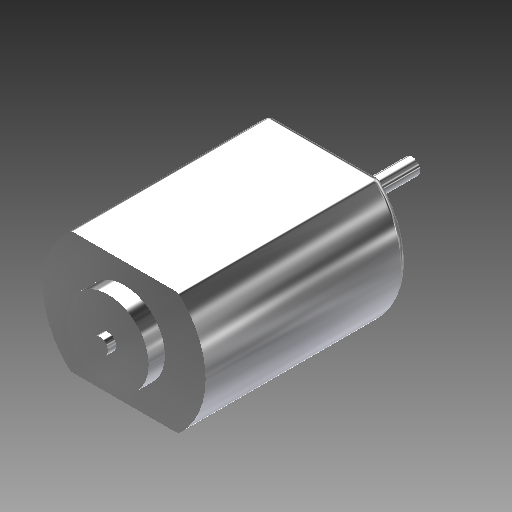
# Autodesk Inventor part: motor
Saved by Autodesk Inventor 2017 (Build 210142000, 142)
## iProperties
Created: 2016-09-08
Part Number: motor
Material: Aluminum 6061
Document SubType Name: Modeling
Designer: Paulo Loma
Density: 2.7 g/cm^3
Appearance: Aluminum - Flat
Author: Paulo Loma
Autodesk Inventor part; units mm, degrees
ref_plane "YZ Plane" through (0, 0, 0) normal (1, 0, 0) x (0, 1, 0)
ref_plane "XZ Plane" through (0, 0, 0) normal (0, 1, 0) x (-1, 0, 0)
ref_plane "XY Plane" through (0, 0, 0) normal (0, 0, 1) x (1, 0, 0)
sketch "Sketch1" plane through (0, 0, 0) normal (0, 0, 1) x (1, 0, 0)
  circle A0 centre (0, 0) radius 1
  dimension "d0" = 2
  constraints: 1 centre point, 1 coincident
  measures "d0" diameter of A0
extrude "Extrusion1" add sketch "Sketch1" along normal blind 8.4
sketch "Sketch2" plane through (0, 0, 8.4) normal (0, 0, 1) x (1, 0, 0)
  circle A0 centre (0, 0) radius 3
  dimension "d3" = 6
  constraints: 1 centre point, 1 coincident
  measures "d3" diameter of A0
extrude "Extrusion2" add sketch "Sketch2" along normal blind 2
sketch "Sketch3" plane through (0, 0, 10.4) normal (0, 0, 1) x (1, 0, 0)
  line L0 (-6.6144, -7.5) -> (6.6144, -7.5)
  line L1 (6.6144, 7.5) -> (-6.6144, 7.5)
  line L2 (-10, -7.5) -> (10, 7.5) construction
  line L3 (10, -7.5) -> (-10, 7.5) construction
  arc A0 (-6.6144, 7.5) -> (-6.6144, -7.5) centre (0, 0) ccw
  arc A1 (6.6144, -7.5) -> (6.6144, 7.5) centre (0, 0) ccw
  constraints: 8 end point, 4 point on circle, 2 centre point, 2 midpoint, 1 coincident, 1 horizontal, 1 parallel
extrude "Extrusion3" add sketch "Sketch3" along normal blind 25
sketch "Sketch4" plane through (0, 0, 35.4) normal (0, 0, 1) x (1, 0, 0)
  arc A0 (2.1794, -4.5) -> (-2.1794, -4.5) centre (0, 0) ccw
  line L0 (0, -4.5) -> (2.1794, -4.5)
  line L1 (0, -4.5) -> (-2.1794, -4.5)
  dimension "d10" = 10
  constraints: 4 end point, 2 point on circle, 1 centre point, 1 coincident, 1 horizontal, 1 point on line
  measures "d10" diameter of A0
extrude "Extrusion4" add sketch "Sketch4" along normal blind 2
sketch "Sketch5" plane through (0, 0, 37.4) normal (0, 0, 1) x (1, 0, 0)
  circle A0 centre (0, 0) radius 1
  dimension "d14" = 2
  constraints: 1 centre point, 1 coincident
  measures "d14" diameter of A0
extrude "Extrusion5" add sketch "Sketch5" along normal blind 1
fillet "Fillet7" radius 1 1 edges at (10, 0, 10.4)
fillet "Fillet8" radius 1 1 edges at (-10, 0, 10.4)
fillet "Fillet9" radius 1 5 edges at (0, -7.5, 10.4) (-6.0606, -7.5, 10.6339) (-6.6144, -7.5, 23.4) (6.0606, -7.5, 10.6339) (6.6144, -7.5, 23.4)
fillet "Fillet10" radius 1 5 edges at (0, 7.5, 10.4) (6.0606, 7.5, 10.6339) (6.6144, 7.5, 23.4) (-6.0606, 7.5, 10.6339) (-6.6144, 7.5, 23.4)
body "Solid1"
